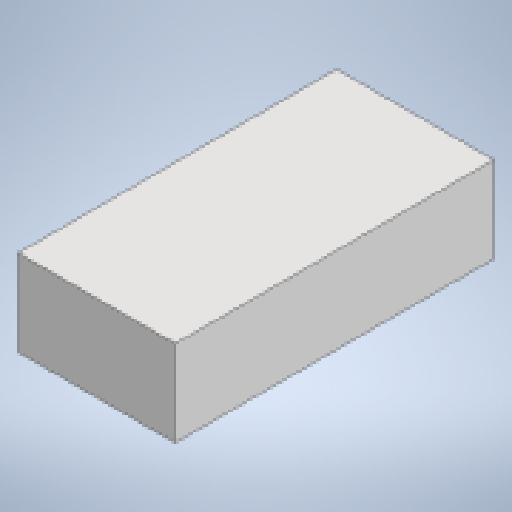
# Autodesk Inventor part: Buck
Saved by Autodesk Inventor 2024 (Build 280153000, 153)
## iProperties
Created: 2024-07-20
Part Number: Buck
Material: Genérico
Document SubType Name: Modeling
Designer: sergi
Density: 1 g/cm^3
Appearance: Valor por defecto
Author: sergi
Autodesk Inventor part; units mm, degrees
ref_plane "YZ Plane" through (0, 0, 0) normal (1, 0, 0) x (0, 1, 0)
ref_plane "XZ Plane" through (0, 0, 0) normal (0, 1, 0) x (-1, 0, 0)
ref_plane "XY Plane" through (0, 0, 0) normal (0, 0, 1) x (1, 0, 0)
sketch "Boceto1" plane through (0, 0, 0) normal (0, 1, 0) x (-1, 0, 0)
  line L0 (-10.7, 21.7) -> (10.7, 21.7)
  line L1 (10.7, 21.7) -> (10.7, -21.7)
  line L2 (10.7, -21.7) -> (-10.7, -21.7)
  line L3 (-10.7, -21.7) -> (-10.7, 21.7)
  line L4 (-10.7, 21.7) -> (10.7, -21.7) construction
  line L5 (10.7, 21.7) -> (-10.7, -21.7) construction
  point P0 (0, 0)
  dimension "d0" = 21.4
  dimension "d1" = 43.4
  constraints: 12 end point, 2 midpoint, 2 parallel, 1 horizontal, 1 perpendicular
  measures "d0" distance of L1.end L2.end
  measures "d1" distance of L0.end L1.end
extrude "Extrusión1" add sketch "Boceto1" along normal blind 11.7
sketch "Boceto2" plane through (0, 11.7, 0) normal (0, 1, 0) x (1, 0, 0)
  line L0 (10.7, 21.7) -> (-10.7, 21.7) projected
  line L1 (-10.7, 21.7) -> (-10.7, -21.7) projected
  line L2 (-10.7, -21.7) -> (10.7, -21.7) projected
  line L3 (10.7, -21.7) -> (10.7, 21.7) projected
  line L4 (-9.7, 20.7) -> (9.7, 20.7)
  line L5 (9.7, 20.7) -> (9.7, -20.7)
  line L6 (9.7, -20.7) -> (-9.7, -20.7)
  line L7 (-9.7, -20.7) -> (-9.7, 20.7)
  line L8 (-6.25, 17.1) -> (9.7, 17.1)
  line L9 (5.95, -17.1) -> (-9.7, -17.1)
  circle A0 centre (8.15, 15.55) radius 1.55
  circle A1 centre (-8.15, -15.55) radius 1.55
  point P0 (0, 0)
  dimension "d4" = 1
  dimension "d5" = 4.6
  dimension "d6" = 3.1
  dimension "d7" = 3.1
  dimension "d8" = 3.6
  constraints: 12 end point, 4 tangent, 2 centre point, 2 point on line, 3 other
  measures "d4" distance between parallel lines of L0 L4
  measures "d5" distance between parallel lines of L0 L8
  measures "d6" diameter of A0
  measures "d7" diameter of A1
  measures "d8" distance between parallel lines of L6 L9
hole "Agujero1" at (8.15, 11.7, -15.55) at (-8.15, 11.7, 15.55) direction (0, -1, 0) diameter 3.1 end through all
